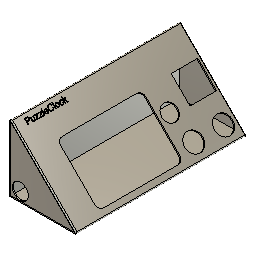
casev2 (Autodesk Fusion 360 design; units mm, degrees)
Autodesk Fusion 360 part; units mm, degrees
note: some values were not read from the file. Set by a fixed rule: which sketch regions a step uses.
sketch "Sketch1" plane through (0, 0, 0) normal (0, 0, 1) x (1, 0, 0)
  line L0 (0, 0) -> (0, 60)
  line L1 (0, 0) -> (60, 0)
  line L2 (-1, -1) -> (63, -1)
  line L3 (-1, 63) -> (-1, -1)
  line L4 (0, 60) -> (60, 0)
  line L5 (-1, 63) -> (63, -1)
  dimension "d2" = 60
  dimension "d3" = 60
  dimension "d4" = 64
  dimension "d5" = 64
  dimension "d6" = 1
  dimension "d7" = 1
  constraint coincident L0.start L1.start
  constraint perpendicular L0 L1
  constraint horizontal L2
  constraint vertical L3
  measures "d2" distance of L0.start L0.end
  measures "d3" distance of L0.start L1.end
  measures "d4" distance of L2.start L2.end
  measures "d5" distance of L2.start L3.start
  measures "d6" distance of L1 L2
  measures "d7" distance of L0 L3
extrude "Extrude1" add sketch "Sketch1" along normal blind 160 makes body 1
sketch "Sketch2" plane through (31, 31, 0) normal (0.707107, 0.707107, 0) x (0, 0, -1)
  line L0 (0, -45.2548) -> (0, 45.2548)
  line L1 (0, 45.2548) -> (-160, 45.2548)
  line L2 (-160, 45.2548) -> (-160, -45.2548)
  line L3 (-160, -45.2548) -> (0, -45.2548)
  line L4 (-130.3693, 17.0756) -> (-60.3693, 17.0756)
  line L5 (-55.3693, 12.0756) -> (-55.3693, -32.9244)
  line L6 (-60.3693, -37.9244) -> (-130.3693, -37.9244)
  line L7 (-135.3693, -32.9244) -> (-135.3693, 12.0756)
  circle A0 centre (-40, -30) radius 8.5
  circle A1 centre (-12, -30) radius 8.5
  circle A2 centre (-45, -5) radius 7.5
  arc A3 (-55.3693, 12.0756) -> (-60.3693, 17.0756) centre (-60.3693, 12.0756) ccw
  arc A4 (-130.3693, 17.0756) -> (-135.3693, 12.0756) centre (-130.3693, 12.0756) ccw
  arc A5 (-135.3693, -32.9244) -> (-130.3693, -37.9244) centre (-130.3693, -32.9244) ccw
  arc A6 (-60.3693, -37.9244) -> (-55.3693, -32.9244) centre (-60.3693, -32.9244) ccw
  line L8 (-150, 30) -> (-110, 30) construction
  line L9 (-110, 30) -> (-110, 40) construction
  line L10 (-110, 40) -> (-150, 40) construction
  line L11 (-150, 40) -> (-150, 30) construction
  line L12 (-28, -8) -> (-3, -8)
  line L13 (-3, -8) -> (-3, 17)
  line L14 (-3, 17) -> (-28, 17)
  line L15 (-28, 17) -> (-28, -8)
  point P0 (-135.3693, 17.0756)
  point P1 (-55.3693, 17.0756)
  point P2 (-135.3693, -37.9244)
  dimension "d10" = 80
  dimension "d11" = 55
  dimension "d12" = 17
  dimension "d13" = 17
  dimension "d14" = 15
  dimension "d16" = 5
  dimension "d17" = 5
  dimension "d18" = 5
  dimension "d19" = 5
  dimension "d20" = 5
  dimension "d32" = 25
  dimension "d33" = 25
  text T0 "PuzzleClock" font "Arial" height 5 align left top in box 40 x 10 at (-150, 30) x (1, 0) y (0, 1) spacing 1
  constraint horizontal L4
  constraint vertical L5
  constraint horizontal L6
  constraint vertical L7
  constraint coincident P1 L4
  constraint coincident P1 L5
  constraint tangent L4 A3
  constraint tangent L5 A3
  constraint coincident P0 L4
  constraint coincident P0 L7
  constraint tangent L4 A4
  constraint tangent L7 A4
  constraint coincident P2 L6
  constraint coincident P2 L7
  constraint tangent L6 A5
  constraint tangent L7 A5
  constraint tangent L6 A6
  constraint tangent L5 A6
  constraint horizontal L12
  constraint vertical L13
  constraint horizontal L14
  constraint vertical L15
  measures "d10" distance of P0 P1
  measures "d11" distance of P0 P2
  measures "d12" diameter of A0
  measures "d13" diameter of A1
  measures "d14" diameter of A2
  measures "d16" radius of A3
  measures "d17" radius of A4
  measures "d18" radius of A5
  measures "d19" radius of A6
  measures "d32" distance of L12.start L12.end
  measures "d33" distance of L12.start L14.end
extrude "Extrude2" cut sketch "Sketch2" against normal blind 0.5 text T0 bodies 1
extrude "Extrude3" cut sketch "Sketch2" against normal blind 5 contours L4 L5 L6 L7 A3 A4 A5 A6 bodies 1
extrude "Extrude4" cut sketch "Sketch2" against normal blind 5 contours A0 | A1 | A2 bodies 1
extrude "Extrude5" add sketch "Sketch1" along normal blind 1 separate body contours L0 L1 L4 makes body 2
extrude "Extrude6" add sketch "Sketch1" along normal blind 1 from surface at 159 separate body contours L0 L1 L4 makes body 3
extrude "Extrude7" cut sketch "Sketch2" against normal blind 10 contours L12 L13 L14 L15 bodies 1
sketch "Sketch3" plane through (0, 0, 160) normal (0, 0, 1) x (1, 0, 0)
  line L0 (0, 0) -> (60, 0)
  line L1 (60, 0) -> (0, 60)
  line L2 (0, 60) -> (0, 0)
  circle A0 centre (9, 8) radius 7.5
  dimension "d36" = 15
  measures "d36" diameter of A0
extrude "Extrude8" cut sketch "Sketch3" against normal blind 5 contours A0 bodies 3
fillet "Fillet1" radius 1 4 edges at (-1, 63, 80) (63, -1, 80) (31, 31, 160) (31, 31, 0) on bodies 1
